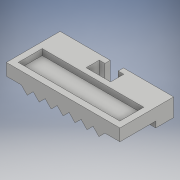
# Autodesk Inventor part: Clamp-part2(moving)-Base9x19mm.
Saved by Autodesk Inventor 2017 (Build 210142000, 142)
## iProperties
Created: 2021-08-04
Part Number: Clamp-part2(moving)-Base9x19mm.
Material: Generic
Document SubType Name: Modeling
Designer: Nikita
Density: 1 g/cm^3
Appearance: Default
Author: Nikita
Autodesk Inventor part; units mm, degrees
ref_plane "YZ Plane" through (0, 0, 0) normal (1, 0, 0) x (0, 1, 0)
ref_plane "XZ Plane" through (0, 0, 0) normal (0, 1, 0) x (-1, 0, 0)
ref_plane "XY Plane" through (0, 0, 0) normal (0, 0, 1) x (1, 0, 0)
sketch "Sketch1" plane through (0, 0, 0) normal (0, 0, 1) x (1, 0, 0)
  line L0 (0, 0) -> (19, 0)
  line L1 (19, 0) -> (19, 9)
  line L2 (19, 9) -> (0, 9)
  line L3 (0, 9) -> (0, 0)
  point P0 (9.5, 9)
  dimension "d0" = 19
  dimension "d1" = 9
  constraints: 8 end point, 2 parallel, 1 horizontal, 1 midpoint, 1 perpendicular
  measures "d0" distance of L2.end L1.end
  measures "d1" distance of L1.end L0.end
extrude "Extrusion1" add sketch "Sketch1" along normal blind 3
sketch "Sketch10" plane through (0, 0, 0) normal (-1, 0, 0) x (0, 0, 1)
  line L0 (0, 0) -> (3, 0) projected
  line L1 (3, 9) -> (3, 0) projected
  line L2 (3, 0) -> (2, 0)
  line L3 (2, 0) -> (2, 6)
  line L4 (2, 6) -> (3, 6)
  line L5 (3, 6) -> (3, 0)
  line L6 (3, 0) -> (2, 1)
  line L7 (3, 0) -> (4.4142, 0) construction
  line L8 (2, 1) -> (3, 2)
  line L9 (3, 0) -> (3, 9) projected
  line L10 (3, 2) -> (2, 3)
  line L11 (2, 3) -> (3, 4)
  line L12 (2, 5) -> (3, 4)
  line L13 (2, 5) -> (3, 5)
  dimension "d23" = 1
  dimension "d24" = 6
  dimension "d25" = 135
  dimension "d26" = 90
  constraints: 22 end point, 5 point on line, 3 perpendicular, 2 horizontal, 2 parallel, 1 equal length, 1 midpoint
  measures "d23" distance of L4.end L3.end
  measures "d24" distance of L2.end L3.end
  measures "d25" angle of L7 L6
  measures "d26" angle of L6 L8
extrude "Extrusion8" cut sketch "Sketch10" against normal up to next contours L6 L8 L1 | L10 L11 L1 | L12 L13 L1 | L3 L4 L1 L13
sketch "Sketch11" plane through (0, 0, 0) normal (0, -1, 0) x (1, 0, 0)
  line L0 (0, 3) -> (19, 3) projected
  line L1 (0, 3) -> (19, 3)
  line L2 (19, 3) -> (19, 2)
  line L3 (19, 2) -> (8.5, 2)
  line L4 (0, 2) -> (0, 3)
  line L5 (0, 3) -> (0, 2) projected
  line L6 (0, 3) -> (1.4142, 3) construction
  line L7 (19, 3) -> (0, 3) projected
  line L8 (9.5, 3) -> (8.5, 2)
  line L9 (9.5, 3) -> (10.9142, 3) construction
  line L10 (10.5, 2) -> (8.5, 2)
  line L11 (9.5, 3) -> (10.5, 2)
  line L12 (10.5, 2) -> (8.5, 2)
  line L13 (8.5, 2) -> (0, 2)
  line L14 (7.5, 3) -> (8.5, 2)
  line L15 (8.5, 2) -> (6.5, 2)
  line L16 (7.5, 3) -> (6.5, 2)
  line L17 (5.5, 3) -> (6.5, 2)
  line L18 (6.5, 2) -> (4.5, 2)
  line L19 (5.5, 3) -> (4.5, 2)
  line L20 (3.5, 3) -> (4.5, 2)
  line L21 (4.5, 2) -> (2.5, 2)
  line L22 (3.5, 3) -> (2.5, 2)
  line L23 (12.5, 2) -> (10.5, 2)
  line L24 (11.5, 3) -> (12.5, 2)
  line L25 (11.5, 3) -> (10.5, 2)
  line L26 (14.5, 2) -> (12.5, 2)
  line L27 (13.5, 3) -> (14.5, 2)
  line L28 (13.5, 3) -> (12.5, 2)
  line L29 (16.5, 2) -> (14.5, 2)
  line L30 (15.5, 3) -> (16.5, 2)
  line L31 (15.5, 3) -> (14.5, 2)
  point P0 (0, 0)
  dimension "d30" = 135
  dimension "d33" = 2
  dimension "d40" = 2
  constraints: 58 end point, 5 horizontal, 5 point on line, 3 collinear, 3 parallel, 2 perpendicular, 1 coincident, 1 equal length, 39 other
  measures "d30" angle of L8 L9
  measures "d33" distance of L8.start L14.start
  measures "d40" distance of L11.end L23.start
extrude "Extrusion9" cut sketch "Sketch11" against normal blind 6 contours L0 L22 L13 L4 | L0 L19 L20 | L0 L16 L17 | L0 L8 L14 | L0 L25 L11 | L0 L28 L24 | L0 L31 L27 | L0 L2 L3 L30
sketch "Sketch12" plane through (0, 0, 3) normal (0, 0, 1) x (1, 0, 0)
  line L0 (19, 9) -> (0, 9) projected
  line L1 (11.5494, 5.9) -> (7.4494, 5.9)
  line L2 (7.4494, 5.9) -> (7.4494, 8.1)
  line L3 (7.4494, 8.1) -> (11.5494, 8.1)
  line L4 (11.5494, 8.1) -> (11.5494, 5.9)
  line L5 (11.5494, 5.9) -> (7.4494, 8.1) construction
  line L6 (7.4494, 5.9) -> (11.5494, 8.1) construction
  line L7 (10.5994, 7.2) -> (8.3994, 7.2)
  line L8 (8.3994, 7.2) -> (8.3994, 9)
  line L9 (8.3994, 9) -> (10.5994, 9)
  line L10 (10.5994, 9) -> (10.5994, 7.2)
  line L11 (10.5994, 7.2) -> (8.3994, 9) construction
  line L12 (8.3994, 7.2) -> (10.5994, 9) construction
  point P0 (0, 0)
  point P1 (9.4994, 7)
  point P2 (9.4994, 8.1)
  dimension "d47" = 2
  dimension "d48" = 4.1
  dimension "d49" = 2.2
  dimension "d50" = 2.2
  constraints: 24 end point, 5 midpoint, 4 parallel, 2 horizontal, 2 perpendicular, 1 point on line
  measures "d47" distance from line of L0 point (9.499, 7)
  measures "d48" distance of L2.end L3.end
  measures "d49" distance of L1.end L2.end
  measures "d50" distance of L8.end L9.end
extrude "Extrusion10" cut sketch "Sketch12" against normal up to next
sketch "Sketch13" plane through (0, 0, 0) normal (0, 0, -1) x (-1, 0, 0)
  line L0 (-8.3994, 9) -> (-8.3994, 8.1) projected
  line L1 (-8.3994, 8.1) -> (-7.4494, 8.1) projected
  line L2 (-7.4494, 8.1) -> (-7.4494, 5.9) projected
  line L3 (-7.4494, 5.9) -> (-11.5494, 5.9) projected
  line L4 (-11.5494, 5.9) -> (-11.5494, 8.1) projected
  line L5 (-11.5494, 8.1) -> (-10.5994, 8.1) projected
  line L6 (-10.5994, 8.1) -> (-10.5994, 9) projected
  line L7 (-19, 9) -> (-10.5994, 9) projected
  line L8 (-19, 0) -> (-19, 9) projected
  line L9 (0, 0) -> (-19, 0) projected
  line L10 (0, 9) -> (0, 0) projected
  line L11 (-8.3994, 9) -> (0, 9) projected
  line L12 (-10.5, 3) -> (-8.5, 3) projected
  line L13 (-1, 5) -> (-18, 5)
  line L14 (-18, 5) -> (-18, 1)
  line L15 (-18, 1) -> (-1, 1)
  line L16 (-1, 1) -> (-1, 5)
  line L17 (-1, 5) -> (-18, 1) construction
  line L18 (-18, 5) -> (-1, 1) construction
  point P0 (-9.5, 3)
  dimension "d53" = 17
  dimension "d54" = 4
  constraints: 12 end point, 3 midpoint, 2 parallel, 1 horizontal, 1 perpendicular
  measures "d53" distance of L15.end L14.end
  measures "d54" distance of L14.end L13.end
extrude "Extrusion11" cut sketch "Sketch13" against normal blind 1 contours L16 L15 L14 L13
sketch "Sketch14" plane through (0, 0, 2) normal (0, 0, 1) x (1, 0, 0)
  line L0 (6.4994, 5) -> (12.4994, 5)
  line L1 (12.4994, 5) -> (12.4994, 6)
  line L2 (12.4994, 6) -> (6.4994, 6)
  line L3 (6.4994, 6) -> (6.4994, 5)
  line L4 (6.4994, 5) -> (12.4994, 6) construction
  line L5 (12.4994, 5) -> (6.4994, 6) construction
  line L6 (19, 9) -> (10.5994, 9) projected
  point P0 (0, 0)
  point P1 (9.4994, 5.5)
  dimension "d57" = 6
  dimension "d58" = 1
  dimension "d59" = 3.5
  constraints: 12 end point, 2 midpoint, 2 parallel, 1 horizontal, 1 perpendicular
  measures "d57" distance of L2.end L1.end
  measures "d58" distance of L1.end L0.end
  measures "d59" distance from line of L6 point (9.499, 5.5)
extrude "Extrusion12" add sketch "Sketch14" along normal blind 1
chamfer "Chamfer1" distance 0.5 angle 45 1 edges at (9.4994, 5, 3)
sketch "WeightSection-5mm" plane through (0, 0, 0) normal (-1, 0, 0) x (0, 0, 1)
  line L0 (0, 5) -> (1, 5) projected
  line L1 (1, 5) -> (1, 1) projected
  line L2 (0, 1) -> (1, 1) projected
  circle A0 centre (-1.5334, 3) radius 2.5
  point P0 (0, 0)
  dimension "d65" = 5
  constraints: 1 centre point
  measures "d65" diameter of A0
body "Solid1"
